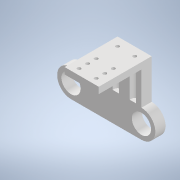
# Autodesk Inventor part: IntakeChainLinkVP
Saved by Autodesk Inventor 2020 (Build 240168000, 168)
## iProperties
Created: 2020-01-19
Part Number: IntakeChainLinkVP
Material: Generic
Document SubType Name: Modeling
Designer: srini
Density: 1 g/cm^3
Appearance: Default
Author: srini
Autodesk Inventor part; units mm, degrees
ref_plane "YZ Plane" through (0, 0, 0) normal (1, 0, 0) x (0, 1, 0)
ref_plane "XZ Plane" through (0, 0, 0) normal (0, 1, 0) x (-1, 0, 0)
sketch "Sketch1" plane through (0, 0, 0) normal (0, 0, 1) x (1, 0, 0)
  line L0 (-52.3875, 0) -> (52.3875, 0) construction
  line L1 (-52.3875, -20.6502) -> (52.3875, -20.6502)
  line L2 (52.3875, 20.6502) -> (-52.3875, 20.6502)
  arc A0 (-52.3875, 20.6502) -> (-52.3875, -20.6502) centre (-52.3875, 0) ccw
  arc A1 (52.3875, -20.6502) -> (52.3875, 20.6502) centre (52.3875, 0) ccw
  point P0 (0, 0)
  dimension "d0" = 104.775
  dimension "d1" = 20.6502
  constraints: 8 end point, 4 point on circle, 4 tangent, 2 centre point, 1 horizontal, 1 midpoint, 1 parallel
  measures "d0" distance of L0.start L0.end
  measures "d1" radius of A0
extrude "Extrusion1" add sketch "Sketch1" along normal blind 15.24
sketch "Sketch2" plane through (0, 0, 15.24) normal (0, 0, 1) x (1, 0, 0)
  arc A0 (-52.3875, 20.6502) -> (-52.3875, -20.6502) centre (-52.3875, 0) ccw projected
  circle A1 centre (-52.3875, 0) radius 14.3002
  arc A2 (52.3875, -20.6502) -> (52.3875, 20.6502) centre (52.3875, 0) ccw projected
  circle A3 centre (52.3875, 0) radius 14.3002
  point P0 (0, 0)
  dimension "d4" = 28.6004
  constraints: 2 centre point, 2 coincident, 1 equal radius
  measures "d4" diameter of A1
extrude "Extrusion2" cut sketch "Sketch2" against normal through all
sketch "Sketch3" plane through (0, 0, 15.24) normal (0, 0, 1) x (1, 0, 0)
  line L0 (1.5875, 79.4246) -> (52.3875, 79.4246)
  line L1 (52.3875, 79.4246) -> (52.3875, 20.6502)
  line L2 (52.3875, 20.6502) -> (1.5875, 20.6502)
  line L3 (1.5875, 20.6502) -> (1.5875, 79.4246)
  line L4 (52.3875, 20.6502) -> (-52.3875, 20.6502) projected
  circle A0 centre (26.9875, 101.6496) radius 7.0281
  circle A1 centre (52.3875, 0) radius 14.3002 projected
  point P0 (0, 0)
  point P1 (26.9875, 20.6502)
  point P2 (26.9875, 79.4246)
  dimension "d7" = 50.8
  dimension "d8" = 22.225
  dimension "d9" = 104.775
  dimension "d10" = 79.4246
  constraints: 8 end point, 2 midpoint, 2 parallel, 1 centre point, 1 collinear, 1 horizontal, 1 perpendicular, 1 point on line, 1 vertical alignment
  measures "d7" distance of L0.start L0.end
  measures "d8" distance from line of A0.centre L0
  measures "d9" distance of A1.centre A0.centre
  measures "d10" distance from line of A1.centre L0
extrude "Extrusion3" add sketch "Sketch3" against normal up to surface (15.24 mm away) contours L0 L1 L2 L3
sketch "Sketch4" plane through (0, 0, 15.24) normal (0, 0, 1) x (1, 0, 0)
  line L0 (1.5875, 79.4246) -> (1.5875, 20.6502) projected
  line L1 (1.5875, 79.4246) -> (52.3875, 79.4246)
  line L2 (52.3875, 79.4246) -> (52.3875, 69.8996)
  line L3 (52.3875, 69.8996) -> (1.5875, 69.8996)
  line L4 (1.5875, 69.8996) -> (1.5875, 79.4246)
  line L5 (52.3875, 20.6502) -> (52.3875, 79.4246) projected
  point P0 (0, 0)
  point P1 (25.4, 20.6502)
  dimension "d13" = 9.525
  constraints: 8 end point, 2 parallel, 1 horizontal, 1 perpendicular, 2 other
  measures "d13" distance of L1.end L2.end
extrude "Extrusion4" add sketch "Sketch4" along normal blind 63.5
sketch "Sketch5" plane through (1.5875, 79.4246, 0) normal (0, 1, 0) x (1, 0, 0)
  circle A0 centre (38.1, -12.7) radius 2.5797
  line L0 (0, 0) -> (50.8, 0) projected
  line L1 (50.8, 0) -> (50.8, -78.74) projected
  circle A1 centre (12.7, -12.7) radius 2.5797
  circle A2 centre (38.1, -44.45) radius 2.5797
  circle A3 centre (12.7, -44.45) radius 2.5797
  circle A4 centre (38.1, -57.15) radius 2.5797
  circle A5 centre (12.7, -57.15) radius 2.5797
  circle A6 centre (38.1, -69.85) radius 2.5797
  circle A7 centre (12.7, -69.85) radius 2.5797
  line L2 (25.4, 0) -> (25.4, -6.0461)
  dimension "d17" = 5.1594
  dimension "d18" = 12.7
  dimension "d21" = 25.4
  dimension "d24" = 31.75
  dimension "d29" = 12.7
  dimension "d51" = 12.7
  constraints: 8 centre point, 3 vertical, 2 end point, 1 horizontal, 1 midpoint, 14 other
  measures "d17" diameter of A0
  measures "d18" distance from line of A0.centre L0
  measures "d21" distance of A0.centre A1.centre
  measures "d24" distance of A0.centre A2.centre
  measures "d29" distance of A2.centre A4.centre
  measures "d51" distance from line of A0.centre L2
extrude "Extrusion5" cut sketch "Sketch5" against normal blind 50.8
ref_plane "Work Plane1" through (1.5875, 73.0746, 0) normal (0, 1, 0) x (1, 0, 0)
sketch "Sketch6" plane through (1.5875, 73.0746, 0) normal (0, 1, 0) x (1, 0, 0)
  line L0 (-53.975, 0) -> (50.8, 0) projected
  line L1 (50.8, -15.24) -> (50.8, -78.74) projected
  line L2 (38.1, -12.7) -> (38.1, -19.05) construction
  line L3 (33.3375, -12.7) -> (33.3375, -19.05)
  line L4 (42.8625, -19.05) -> (42.8625, -12.7)
  arc A0 (42.8625, -12.7) -> (33.3375, -12.7) centre (38.1, -12.7) ccw
  arc A1 (33.3375, -19.05) -> (42.8625, -19.05) centre (38.1, -19.05) ccw
  line L5 (12.7, -12.7) -> (12.7, -19.05) construction
  line L6 (7.9375, -12.7) -> (7.9375, -19.05)
  line L7 (17.4625, -19.05) -> (17.4625, -12.7)
  arc A2 (17.4625, -12.7) -> (7.9375, -12.7) centre (12.7, -12.7) ccw
  arc A3 (7.9375, -19.05) -> (17.4625, -19.05) centre (12.7, -19.05) ccw
  circle A4 centre (38.1, -44.45) radius 2.5797 construction
  circle A5 centre (38.1, -69.85) radius 2.5797 construction
  line L8 (38.1, -44.45) -> (38.1, -69.85) construction
  line L9 (33.3375, -44.45) -> (33.3375, -69.85)
  line L10 (42.8625, -69.85) -> (42.8625, -44.45)
  arc A6 (42.8625, -44.45) -> (33.3375, -44.45) centre (38.1, -44.45) ccw
  arc A7 (33.3375, -69.85) -> (42.8625, -69.85) centre (38.1, -69.85) ccw
  circle A8 centre (12.7, -44.45) radius 2.5797 construction
  circle A9 centre (12.7, -69.85) radius 2.5797 construction
  line L11 (12.7, -44.45) -> (12.7, -69.85) construction
  line L12 (7.9375, -44.45) -> (7.9375, -69.85)
  line L13 (17.4625, -69.85) -> (17.4625, -44.45)
  arc A10 (17.4625, -44.45) -> (7.9375, -44.45) centre (12.7, -44.45) ccw
  arc A11 (7.9375, -69.85) -> (17.4625, -69.85) centre (12.7, -69.85) ccw
  circle A12 centre (38.1, -12.7) radius 2.5797 construction
  circle A13 centre (12.7, -12.7) radius 2.5797 construction
  point P0 (-1.5875, 0)
  point P1 (38.1, -15.875)
  point P2 (12.7, -15.875)
  point P3 (38.1, -57.15)
  point P4 (12.7, -57.15)
  dimension "d47" = 6.35
  dimension "d48" = 4.7625
  constraints: 32 end point, 16 point on circle, 16 tangent, 8 centre point, 8 parallel, 4 midpoint, 3 equal radius, 2 concentric, 1 vertical
  measures "d47" distance of L2.start L2.end
  measures "d48" radius of A1
extrude "Extrusion6" cut sketch "Sketch6" against normal blind 50.8
body "Solid1"
